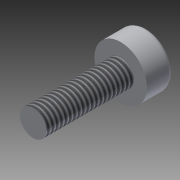
# Autodesk Inventor part: M3_10
Saved by Autodesk Inventor 2013 (Build 170138000, 138)
## iProperties
Created: 2012-10-27
Part Number: M3_10
Document SubType Name: Modeling
Designer: arihon
Density: 2.71 g/cm^3
Material: アルミニウム 6061
Mass: 0.387107 g
Surface Area: 2.21189 cm^2
Volume: 0.142844 cm^3
Author: arihon
Autodesk Inventor part; units mm, degrees
ref_plane "YZ Plane" through (0, 0, 0) normal (1, 0, 0) x (0, 1, 0)
ref_plane "XZ Plane" through (0, 0, 0) normal (0, 1, 0) x (-1, 0, 0)
ref_plane "XY Plane" through (0, 0, 0) normal (0, 0, 1) x (1, 0, 0)
sketch "スケッチ1" plane through (0, 0, 0) normal (0, 0, 1) x (1, 0, 0)
  line L0 (-3, -0.3147) -> (0, -0.3147)
  line L1 (0, -0.3147) -> (0, -3.3147)
  line L2 (0, -3.3147) -> (-3, -3.3147)
  line L3 (-3, -3.3147) -> (-3, -0.3147)
  line L4 (-1.5, -3.3147) -> (0, -3.3147)
  line L5 (0, -3.3147) -> (0, -13.3147)
  line L6 (0, -13.3147) -> (-1.5, -13.3147)
  line L7 (-1.5, -13.3147) -> (-1.5, -3.3147)
  point P0 (0, 0)
  dimension "d0" = 1.5
  dimension "d1" = 0
  dimension "d2" = 10
  dimension "d3" = 0
  dimension "d4" = 3
  constraints: 16 end point, 4 parallel, 2 horizontal, 2 perpendicular, 1 midpoint
  measures "d0" distance between parallel lines of L5 L7
  measures "d1" distance from line of point (0, 0) L5
  measures "d2" distance of L6.end L4.start
  measures "d3" distance from line of point (0, 0) L1
  measures "d4" distance of L2.end L0.start
revolve "回転1" add sketch "スケッチ1" angle 360 about axis through (0, -3.3147, 0) along (0, -1, 0)
thread "ねじ1" size "M3x0.5" class "6g" standard "ANSI Metric M Profile" full length
sketch "スケッチ2" plane through (0, -0.3147, 0) normal (0, 1, 0) x (1, 0, 0)
  circle A0 centre (0, 0) radius 3 projected
  line L0 (0, 1.5) -> (1.299, 0.75)
  line L1 (1.299, 0.75) -> (1.299, -0.75)
  line L2 (1.299, -0.75) -> (0, -1.5)
  line L3 (0, -1.5) -> (-1.299, -0.75)
  line L4 (-1.299, -0.75) -> (-1.299, 0.75)
  line L5 (-1.299, 0.75) -> (0, 1.5)
  dimension "d8" = 1.5
  constraints: 12 end point, 1 coincident, 13 other
  measures "d8" distance of point (0, 0) L0.start
extrude "押し出し1" cut sketch "スケッチ2" against normal blind 2 contours L0 L1 L2 L3 L4 L5
fillet "フィレット1" radius 0.5 1 edges at (3, -0.3147, 0)
